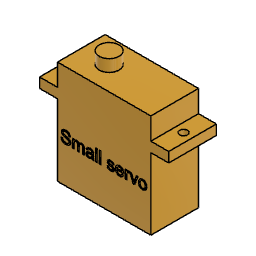
Wrist Exo v4 v7 (Autodesk Fusion 360 archive; units mm, degrees)
design "Small servo"
Autodesk Fusion 360 part; units mm, degrees
sketch "Main body" plane through (0, 0, 0) normal (0, 0, 1) x (1, 0, 0)
  line L0 (0, 0) -> (23.5, 0)
  line L1 (23.5, 0) -> (23.5, 12)
  line L2 (23.5, 12) -> (0, 12)
  line L3 (0, 12) -> (0, 0)
  dimension "d1" = 23.5
  dimension "d2" = 12
  constraint horizontal L0
  constraint vertical L1
  constraint horizontal L2
  constraint vertical L3
  constraint coincident L0.start L3.end
  measures "d1" distance of L0.start L0.end
  measures "d2" distance of L0.start L2.end
extrude "Extrude1" add sketch "Main body" along normal blind 26
sketch "Horn base" plane through (0, 0, 26) normal (0, 0, 1) x (-1, 0, 0)
  line L0 (0, -12) -> (0, 0)
  line L1 (0, 0) -> (-23.5, 0)
  line L2 (-23.5, 0) -> (-23.5, -12)
  line L3 (-23.5, -12) -> (0, -12)
  circle A0 centre (-7, -6) radius 2.5
  dimension "d5" = 5
  dimension "d6" = 6
  dimension "d7" = 7
  measures "d5" diameter of A0
  measures "d6" distance of L3 A0.centre
  measures "d7" distance of L0 A0.centre
extrude "Extrude2" add sketch "Horn base" along normal blind 3 contours A0
sketch "Wing1" plane through (23.5, 0, 0) normal (1, 0, 0) x (0, 1, 0)
  line L0 (0, 0) -> (12, 0)
  line L1 (12, 0) -> (12, 26)
  line L2 (12, 26) -> (0, 26)
  line L3 (0, 26) -> (0, 0)
  line L4 (0, 20.5) -> (12, 20.5)
  line L5 (12, 20.5) -> (12, 18)
  line L6 (12, 18) -> (0, 18)
  line L7 (0, 18) -> (0, 20.5)
  dimension "d10" = 18
  dimension "d11" = 2.5
  constraint horizontal L4
  constraint vertical L5
  constraint horizontal L6
  constraint vertical L7
  constraint coincident L1 L5.end
  constraint coincident L3 L4.start
  measures "d10" distance of L0 L6
  measures "d11" distance of L4 L6
extrude "Wing1 (1)" add sketch "Wing1" along normal blind 4.5 contours L1 L3 L4 L5 L6 L7
sketch "Wing2" plane through (0, 0, 0) normal (-1, 0, 0) x (0, -1, 0)
  line L0 (-12, 0) -> (0, 0)
  line L1 (0, 0) -> (0, 26)
  line L2 (0, 26) -> (-12, 26)
  line L3 (-12, 26) -> (-12, 0)
  line L4 (-12, 20.5) -> (0, 20.5)
  line L5 (0, 20.5) -> (0, 18)
  line L6 (0, 18) -> (-12, 18)
  line L7 (-12, 18) -> (-12, 20.5)
  dimension "d14" = 18
  dimension "d15" = 2.5
  constraint horizontal L4
  constraint vertical L5
  constraint horizontal L6
  constraint vertical L7
  constraint coincident L1 L5.end
  constraint coincident L3 L4.start
  measures "d14" distance of L0 L6
  measures "d15" distance of L4 L6
extrude "Wing2 (1)" add sketch "Wing2" along normal blind 4.5 contours L1 L3 L4 L5 L6 L7
sketch "Holes" plane through (0, 0, 20.5) normal (0, 0, 1) x (-1, 0, 0)
  line L0 (-23.5, -12) -> (-23.5, 0)
  line L1 (-23.5, 0) -> (-28, 0)
  line L2 (-28, 0) -> (-28, -12)
  line L3 (-28, -12) -> (-23.5, -12)
  circle A0 centre (-25.75, -6) radius 1
  circle A1 centre (2.25, -6) radius 1
  line L4 (-11.75, -21) -> (-11.75, 10) construction
  line L5 (0, 0) -> (4.5, 0) construction
  dimension "d18" = 2
  dimension "d19" = 6
  dimension "d20" = 2
  dimension "d21" = 28
  dimension "d22" = 11.75
  dimension "d23" = 14
  dimension "d24" = 6
  constraint vertical L4
  measures "d18" diameter of A0
  measures "d19" distance of L1 A0.centre
  measures "d20" diameter of A1
  measures "d21" horizontal distance of A0.centre A1.centre
  measures "d22" distance of L0 L4
  measures "d23" distance of A0.centre L4
  measures "d24" distance of A1.centre L5
hole "Hole1" at (25.75, 6, 20.5) at (-2.25, 6, 20.5) direction (0, 0, -1) diameter 2 end up to surface (2.5 mm away)
sketch "Text" plane through (0, 0, 0) normal (0, -1, 0) x (1, 0, 0)
  line L0 (0, 0) -> (23.5, 0)
  line L1 (23.5, 0) -> (23.5, 18)
  line L2 (23.5, 18) -> (28, 18)
  line L3 (28, 18) -> (28, 20.5)
  line L4 (28, 20.5) -> (23.5, 20.5)
  line L5 (23.5, 20.5) -> (23.5, 26)
  line L6 (23.5, 26) -> (0, 26)
  line L7 (0, 26) -> (0, 20.5)
  line L8 (0, 20.5) -> (-4.5, 20.5)
  line L9 (-4.5, 20.5) -> (-4.5, 18)
  line L10 (-4.5, 18) -> (0, 18)
  line L11 (0, 18) -> (0, 0)
  line L12 (0.8854, 7.9821) -> (33.8378, 7.6579) construction
  line L13 (33.8378, 7.6579) -> (33.8788, 11.8265) construction
  line L14 (33.8788, 11.8265) -> (0.9264, 12.1507) construction
  line L15 (0.9264, 12.1507) -> (0.8854, 7.9821) construction
  dimension "d28" = 3
  text T0 "Small servo" font "Arial" height 3 align left top in box 32.954 x 4.1688 at (0.8854, 7.9821) x (0.999952, -0.009837) y (0.009837, 0.999952) spacing 1 kerned
extrude "Extrude5" cut sketch "Text" against normal blind 1 text T0

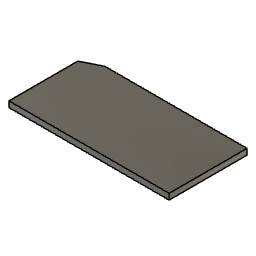
design "Wrist Exo Top Lid"
Autodesk Fusion 360 part; units mm, degrees
sketch "Sketch1" plane through (0, 0, 0) normal (0, 0, 1) x (1, 0, 0)
  line L0 (0, 0) -> (54.5, 0)
  line L1 (54.5, 0) -> (54.5, 26.5)
  line L2 (54.5, 26.5) -> (6.193, 26.5)
  line L3 (6.193, 26.5) -> (0, 23.416)
  line L4 (0, 23.416) -> (0, 0)
  dimension "d3" = 26.5
  dimension "d4" = 54.5
  constraint coincident L0.start L4.end
  constraint horizontal L0
  constraint perpendicular L0 L1
  constraint perpendicular L1 L2
  measures "d3" distance of L0.end L1.end
  measures "d4" distance of L0.start L0.end
extrude "Extrude1" add sketch "Sketch1" along normal blind 2

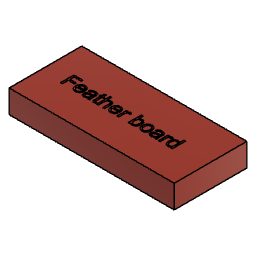
design "Feather board"
Autodesk Fusion 360 part; units mm, degrees
sketch "Sketch1" plane through (0, 0, 0) normal (0, 0, 1) x (1, 0, 0)
  line L0 (0, 0) -> (50, 0)
  line L1 (50, 0) -> (50, 22)
  line L2 (50, 22) -> (0, 22)
  line L3 (0, 22) -> (0, 0)
  dimension "d1" = 50
  dimension "d2" = 22
  constraint horizontal L0
  constraint vertical L1
  constraint horizontal L2
  constraint vertical L3
  constraint coincident L0.start L3.end
  measures "d1" distance of L0.start L0.end
  measures "d2" distance of L0.start L2.end
extrude "Extrude1" add sketch "Sketch1" along normal blind 7
sketch "Sketch3" plane through (0, 0, 7) normal (0, 0, 1) x (-1, 0, 0)
  line L0 (0, -22) -> (0, 0)
  line L1 (0, 0) -> (-50, 0)
  line L2 (-50, 0) -> (-50, -22)
  line L3 (-50, -22) -> (0, -22)
  line L4 (-6.3934, -9.8568) -> (-49.9798, -9.3295) construction
  line L5 (-49.9798, -9.3295) -> (-50.0202, -12.6705) construction
  line L6 (-50.0202, -12.6705) -> (-6.4338, -13.1978) construction
  line L7 (-6.4338, -13.1978) -> (-6.3934, -9.8568) construction
  dimension "d5" = 4
  text T0 "Feather board" font "Arial" height 4 align left top in box 43.5896 x 3.3413 at (-6.3934, -9.8568) x (-0.999927, 0.012098) y (-0.012098, -0.999927) spacing 1 kerned
  constraint midpoint L2
extrude "Extrude2" cut sketch "Sketch3" against normal blind 1 text T0

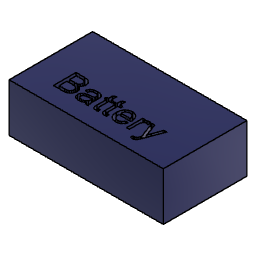
design "Battery 9V"
Autodesk Fusion 360 part; units mm, degrees
sketch "Sketch1" plane through (0, 0, 0) normal (0, 0, 1) x (1, 0, 0)
  line L0 (0, 0) -> (48, 0)
  line L1 (48, 0) -> (48, 26)
  line L2 (48, 26) -> (0, 26)
  line L3 (0, 26) -> (0, 0)
  dimension "d1" = 48
  dimension "d2" = 26
  constraint horizontal L0
  constraint vertical L1
  constraint horizontal L2
  constraint vertical L3
  constraint coincident L0.start L3.end
  measures "d1" distance of L0.start L0.end
  measures "d2" distance of L0.start L2.end
extrude "Extrude1" add sketch "Sketch1" along normal blind 15
sketch "Text" plane through (0, 0, 15) normal (0, 0, 1) x (-1, 0, 0)
  line L0 (0, -26) -> (0, 0)
  line L1 (0, 0) -> (-48, 0)
  line L2 (-48, 0) -> (-48, -26)
  line L3 (-48, -26) -> (0, -26)
  line L4 (-8.4412, -5.8676) -> (-43.5652, -5.8676) construction
  line L5 (-43.5652, -5.8676) -> (-43.5652, -12.3721) construction
  line L6 (-43.5652, -12.3721) -> (-8.4412, -12.3721) construction
  line L7 (-8.4412, -12.3721) -> (-8.4412, -5.8676) construction
  dimension "d5" = 7
  text T0 "Battery" font "Arial" height 7 align left top in box 35.124 x 6.5045 at (-8.4412, -5.8676) x (-1, 0) y (0, -1) spacing 1 kerned
extrude "Extrude2" cut sketch "Text" against normal blind 2 text T0
